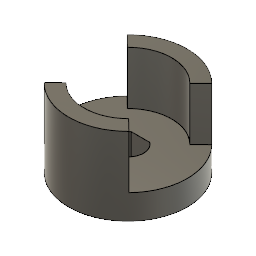
Adaptador_Helice (Autodesk Fusion 360 design; units mm, degrees)
Autodesk Fusion 360 part; units mm, degrees
sketch "Sketch1" plane through (0, 0, 0) normal (0, 1, 0) x (1, 0, 0)
  arc A0 (-1.5, 2) -> (1.5, 2) centre (0, 0) ccw
  line L0 (1.5, 2) -> (-1.5, 2)
  circle A1 centre (0, 0) radius 9.5
  dimension "d1" = 3
  dimension "d2" = 2.5
  dimension "d3" = 19
  constraint coincident A0.centre A1.centre
  constraint horizontal A0.start A0.end
  measures "d1" distance of A0.start A0.end
  measures "d2" radius of A0
  measures "d3" diameter of A1
extrude "Extrude1" add sketch "Sketch1" along normal blind 4
sketch "Sketch2" plane through (0, 4, 0) normal (0, 1, 0) x (-1, 0, 0)
  arc A0 (1.5, -2) -> (-1.5, -2) centre (0, 0) ccw
  line L0 (1.5, -2) -> (-1.5, -2)
  line L1 (4.5, -7) -> (-4.5, -7) construction
  line L2 (0, -14.5329) -> (0, 17.7812) construction
  circle A1 centre (0, 0) radius 9.5 construction
  circle A2 centre (0, 0) radius 7 construction
  line L3 (6.7857, -6.6486) -> (5, -4.899)
  line L4 (-5, -4.899) -> (-6.7857, -6.6486)
  arc A3 (-5, -4.899) -> (5, -4.899) centre (0, 0) ccw
  arc A4 (-6.7857, -6.6486) -> (6.7857, -6.6486) centre (0, 0) ccw
  dimension "d6" = 3
  dimension "d7" = 2.5
  dimension "d8" = 9
  dimension "d9" = 4.5
  dimension "d10" = 14
  dimension "d14" = 10
  dimension "d15" = 7
  dimension "d16" = 9.5
  constraint coincident A0.centre A1.centre
  constraint horizontal L0
  constraint horizontal L1
  constraint coincident A0.centre L2
  constraint vertical L2
  constraint concentric A0 A2
  constraint tangent L1 A2
  constraint coincident A1 L3.start
  constraint coincident A2 L3.end
  constraint coincident A2 L4.start
  constraint coincident A1 L4.end
  constraint collinear A0.centre L4.start L4.end
  constraint collinear A0.centre L3.start L3.end
  constraint horizontal L3.end L4.start
  measures "d6" distance of A0.start A0.end
  measures "d7" radius of A0
  measures "d8" distance of L1.start L1.end
  measures "d9" distance of L1.end L2
  measures "d10" diameter of A2
  measures "d14" horizontal distance of L3.end L4.start
  measures "d15" radius of A3
  measures "d16" radius of A4
extrude "Extrude2" add sketch "Sketch2" along normal blind 8.5 contours L3 L4 A3 A4
mirror "Mirror1" about plane through (0, 0, 0) normal (0, 0, 1) of "Extrude2"
